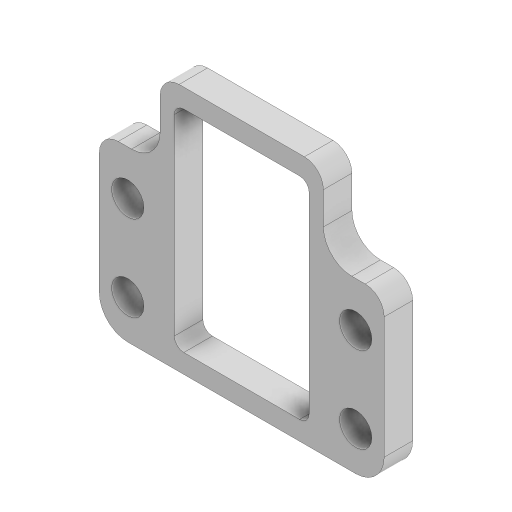
# Autodesk Inventor part: skye_airspeed_inside_back
Saved by Autodesk Inventor 2023 (Build 270158000, 158)
## iProperties
Created: 2023-06-14
Part Number: skye_airspeed_inside_back
Material: Generic
Document SubType Name: Modeling
Designer: Thomas
Density: 1 g/cm^3
Appearance: Default
Author: Thomas
Autodesk Inventor part; units mm, degrees
ref_plane "YZ Plane" through (0, 0, 0) normal (1, 0, 0) x (0, 1, 0)
ref_plane "XZ Plane" through (0, 0, 0) normal (0, 1, 0) x (-1, 0, 0)
ref_plane "XY Plane" through (0, 0, 0) normal (0, 0, 1) x (1, 0, 0)
sketch "Sketch1" plane through (0, 0, 0) normal (0, 0, 1) x (1, 0, 0)
  line L0 (-6.1, 11.1) -> (6.1, 11.1)
  line L1 (7.1, 10.1) -> (7.1, -10.1)
  line L2 (6.1, -11.1) -> (-6.1, -11.1)
  line L3 (-7.1, -10.1) -> (-7.1, 10.1)
  arc A0 (-7.1, -10.1) -> (-6.1, -11.1) centre (-6.1, -10.1) ccw
  arc A1 (6.1, -11.1) -> (7.1, -10.1) centre (6.1, -10.1) ccw
  arc A2 (7.1, 10.1) -> (6.1, 11.1) centre (6.1, 10.1) ccw
  arc A3 (-6.1, 11.1) -> (-7.1, 10.1) centre (-6.1, 10.1) ccw
  circle A4 centre (-12, 0) radius 1.7
  circle A5 centre (-12, -9) radius 1.7
  circle A6 centre (12, 0) radius 1.7
  circle A7 centre (12, -9) radius 1.7
  line L4 (-12, 13.1) -> (6.6, 13.1)
  line L5 (15, 2.7) -> (15, -10.1)
  line L6 (12, -13.1) -> (-12, -13.1)
  line L7 (-15, -10.1) -> (-15, 10.1)
  arc A8 (-12, 13.1) -> (-15, 10.1) centre (-12, 10.1) ccw
  arc A9 (15, 10.1) -> (12, 13.1) centre (12, 10.1) ccw
  arc A10 (12, -13.1) -> (15, -10.1) centre (12, -10.1) ccw
  arc A11 (-15, -10.1) -> (-12, -13.1) centre (-12, -10.1) ccw
  line L8 (8.6, 13.1) -> (15, 13.1)
  line L9 (15, 13.1) -> (15, 4.7)
  line L10 (13, 4.7) -> (11.6, 4.7)
  line L11 (8.6, 7.7) -> (8.6, 11.1)
  arc A12 (8.6, 7.7) -> (11.6, 4.7) centre (11.6, 7.7) ccw
  arc A13 (8.6, 11.1) -> (6.6, 13.1) centre (6.6, 11.1) ccw
  arc A14 (15, 2.7) -> (13, 4.7) centre (13, 2.7) ccw
  line L12 (0, 11.1) -> (0, -11.1) construction
  line L13 (-13, 4.7) -> (-11.6, 4.7)
  line L14 (-8.6, 7.7) -> (-8.6, 11.1)
  arc A15 (-11.6, 4.7) -> (-8.6, 7.7) centre (-11.6, 7.7) ccw
  arc A16 (-6.6, 13.1) -> (-8.6, 11.1) centre (-6.6, 11.1) ccw
  arc A17 (-13, 4.7) -> (-15, 2.7) centre (-13, 2.7) ccw
  point P0 (0, 0)
  point P1 (7.1, -11.1)
  point P2 (7.1, 11.1)
  point P3 (-7.1, -11.1)
  point P4 (-6.6, 13.1)
  dimension "d0" = 14.2
  dimension "d1" = 22.2
  dimension "d2" = 1
  dimension "d3" = 7.1
  dimension "d4" = 11.1
  dimension "d5" = 3.4
  dimension "d8" = 9
  dimension "d11" = 24
  dimension "d14" = 0
  dimension "d15" = 12
  dimension "d16" = 3
  dimension "d17" = 3
  dimension "d18" = 2
  dimension "d19" = 2
  dimension "d20" = 3
  dimension "d23" = 1.5
  dimension "d24" = 3
  dimension "d25" = 3
  dimension "d26" = 2
  constraints: 30 end point, 28 point on circle, 22 tangent, 18 centre point, 12 point on line, 9 symmetric about line, 7 equal radius, 6 parallel, 4 horizontal, 3 perpendicular, 2 midpoint, 1 vertical, 9 other
  measures "d0" distance of point (7.1, -11.1) point (-7.1, -11.1)
  measures "d1" distance of point (7.1, 11.1) point (7.1, -11.1)
  measures "d2" radius of A0
  measures "d3" distance from line of point (0, 0) L3
  measures "d4" distance from line of point (0, 0) L2
  measures "d5" diameter of A4
  measures "d8" distance of A4.centre A5.centre
  measures "d11" distance of A4.centre A6.centre
  measures "d14" vertical distance of point (0, 0) A4.centre
  measures "d15" distance of point (0, 0) A4.centre
  measures "d16" distance from line of L7 A4.centre
  measures "d17" distance from line of L5 A6.centre
  measures "d18" distance between parallel lines of L0 L4
  measures "d19" distance between parallel lines of L2 L6
  measures "d20" radius of A8
  measures "d23" distance between parallel lines of L1 L11
  measures "d24" distance edge to line of A6 L10
  measures "d25" radius of A12
  measures "d26" radius of A13
extrude "Extrusion1" add sketch "Sketch1" along normal blind 3 contours L4 A13 L11 A12 L10 A14 L5 A10 L6 A11 L7 A17 L13 A15 L14 A16
equation "\"d3\" = 0.5 * d0"
equation "\"d4\" = 0.5 * d1"
equation "\"d15\" = 0.5 * d11"
equation "\"d17\" = d16"
body "Solid1"
